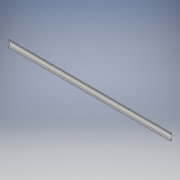
# Autodesk Inventor part: 鋁軌
Saved by Autodesk Inventor 2019 (Build 230136000, 136)
## iProperties
Created: 2018-08-23
Part Number: 鋁軌
Material: 一般
Document SubType Name: Modeling
Designer: elecjack
Density: 1 g/cm^3
Appearance: 預設
Author: elecjack
Autodesk Inventor part; units mm, degrees
ref_plane "YZ Plane" through (0, 0, 0) normal (1, 0, 0) x (0, 1, 0)
ref_plane "XZ Plane" through (0, 0, 0) normal (0, 1, 0) x (-1, 0, 0)
ref_plane "XY Plane" through (0, 0, 0) normal (0, 0, 1) x (1, 0, 0)
sketch "草圖1" plane through (0, 0, 0) normal (0, 0, 1) x (1, 0, 0)
  line L0 (-425, 17.5) -> (425, 17.5)
  line L1 (425, 17.5) -> (425, -17.5)
  line L2 (425, -17.5) -> (-425, -17.5)
  line L3 (-425, -17.5) -> (-425, 17.5)
  point P0 (0, 0)
  dimension "d0" = 850
  dimension "d1" = 35
  dimension "d2" = 17.5
  dimension "d3" = 425
  constraints: 8 end point, 2 parallel, 1 horizontal, 1 perpendicular
  measures "d0" distance between parallel lines of L1 L3
  measures "d1" distance between parallel lines of L2 L0
  measures "d2" distance from line of point (0, 0) L2
  measures "d3" distance from line of point (0, 0) L3
extrude "擠出1" add sketch "草圖1" along normal blind 7.5
sketch "草圖2" plane through (425, -17.5, 0) normal (1, 0, 0) x (0, 0, -1)
  line L0 (0, 35) -> (-7.5, 35) projected
  line L1 (0, 0) -> (0, 35) projected
  line L2 (-6, 35) -> (0, 35)
  line L3 (0, 35) -> (0, 32)
  line L4 (0, 32) -> (-6, 32)
  line L5 (-6, 32) -> (-6, 35)
  line L6 (-6, 3) -> (0, 3)
  line L7 (0, 3) -> (0, 0)
  line L8 (0, 0) -> (-6, 0)
  line L9 (-6, 0) -> (-6, 3)
  line L10 (-7.5, 35) -> (-7.5, 0) projected
  line L11 (-7.5, 30.5) -> (-1, 30.5)
  line L12 (-1, 30.5) -> (-1, 4.5)
  line L13 (-1, 4.5) -> (-7.5, 4.5)
  line L14 (-7.5, 4.5) -> (-7.5, 30.5)
  point P0 (0, 17.5)
  dimension "d6" = 6
  dimension "d7" = 3
  dimension "d8" = 26
  dimension "d9" = 1
  dimension "d10" = 13
  constraints: 24 end point, 6 parallel, 3 horizontal, 3 perpendicular, 3 point on line
  measures "d6" distance between parallel lines of L1 L5
  measures "d7" distance between parallel lines of L4 L0
  measures "d8" distance between parallel lines of L13 L11
  measures "d9" distance between parallel lines of L12 L1
  measures "d10" distance from line of point (0, 17.5) L13
extrude "擠出2" cut sketch "草圖2" against normal blind 850
